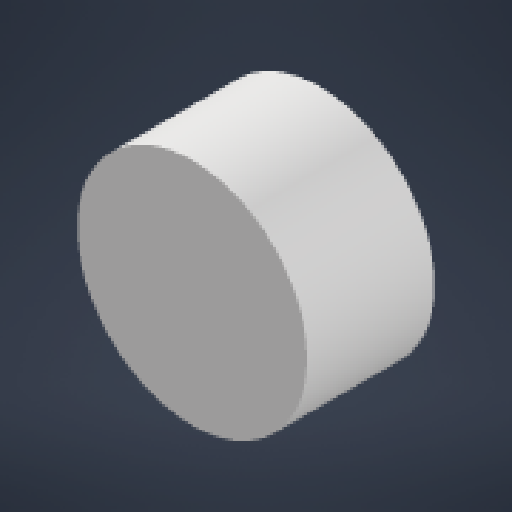
# Autodesk Inventor part: 60mm Wheel Rim
Saved by Autodesk Inventor 2024 (Build 280153000, 153)
## iProperties
Created: 2023-09-10
Part Number: 60mm Wheel Rim
Material: Generic
Document SubType Name: Modeling
Designer: izack
Density: 1 g/cm^3
Appearance: Default
Author: izack
Autodesk Inventor part; units mm, degrees
ref_plane "YZ Plane" through (0, 0, 0) normal (1, 0, 0) x (0, 1, 0)
ref_plane "XZ Plane" through (0, 0, 0) normal (0, 1, 0) x (-1, 0, 0)
ref_plane "XY Plane" through (0, 0, 0) normal (0, 0, 1) x (1, 0, 0)
sketch "Sketch1" plane through (0, 0, 0) normal (0, 0, 1) x (1, 0, 0)
  circle A0 centre (0, 0) radius 22.888
  dimension "d0" = 45.776
  constraints: 1 centre point, 1 coincident
  measures "d0" diameter of A0
extrude "Extrusion1" add sketch "Sketch1" along normal blind 25.4
sketch "Sketch2" plane through (0, 0, 25.4) normal (0, 0, 1) x (1, 0, 0)
  circle A0 centre (0, 0) radius 2.6 construction
  line L0 (1.5011, 2.6) -> (3.0022, 0)
  line L1 (3.0022, 0) -> (1.5011, -2.6)
  line L2 (1.5011, -2.6) -> (-1.5011, -2.6)
  line L3 (-1.5011, -2.6) -> (-3.0022, 0)
  line L4 (-3.0022, 0) -> (-1.5011, 2.6)
  line L5 (-1.5011, 2.6) -> (1.5011, 2.6)
  point P0 (0, 2.6)
  dimension "d3" = 5.2
  constraints: 12 end point, 2 coincident, 1 midpoint, 1 vertical alignment, 15 other
extrude "Extrusion2" cut sketch "Sketch2" against normal blind 25.4
body "Solid1"
